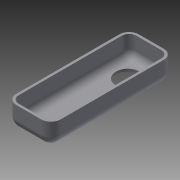
# Autodesk Inventor part: NodeMCU_MQ-4_top_shelled
Saved by Autodesk Inventor 2014 SP1 (Build 180222100, 222)
## iProperties
Created: 2016-10-27
Part Number: NodeMCU_MQ-4_top_shelled
Material: Generic
Document SubType Name: Modeling
Designer: danielsikar
Density: 1 g/cm^3
Appearance: Default
Author: danielsikar
Autodesk Inventor part; units mm, degrees
ref_plane "YZ Plane" through (0, 0, 0) normal (1, 0, 0) x (0, 1, 0)
ref_plane "XZ Plane" through (0, 0, 0) normal (0, 1, 0) x (-1, 0, 0)
ref_plane "XY Plane" through (0, 0, 0) normal (0, 0, 1) x (1, 0, 0)
sketch "Sketch1" plane through (0, 0, 0) normal (0, 0, 1) x (1, 0, 0)
  line L0 (0, 0) -> (37, 0)
  line L1 (37, 0) -> (37, 102.3)
  line L2 (37, 102.3) -> (0, 102.3)
  line L3 (0, 102.3) -> (0, 0)
  dimension "d0" = 37
  dimension "d1" = 102.3
  constraints: 8 end point, 2 parallel, 1 horizontal, 1 perpendicular
  measures "d0" distance of L2.end L1.end
  measures "d1" distance of L1.end L0.end
extrude "Extrusion1" add sketch "Sketch1" along normal blind 19
fillet "Fillet1" radius 8 4 edges at (0, 0, 9.5) (37, 0, 9.5) (37, 102.3, 9.5) (0, 102.3, 9.5)
fillet "Fillet2" radius 8 8 edges at (34.6569, 99.9569, 0) (18.5, 102.3, 0) (2.3431, 99.9569, 0) (0, 51.15, 0) (2.3431, 2.3431, 0) (18.5, 0, 0) (34.6569, 2.3431, 0) (37, 51.15, 0)
shell "Shell1" thickness 2 removed faces 1 at (12.3333, 36.7667, 19)
sketch "Sketch2" plane through (0, 0, 0) normal (0, 0, -1) x (-1, 0, 0)
  circle A0 centre (-18.5, 82.8) radius 10
  line L0 (-8, 102.3) -> (-29, 102.3) projected
  point P0 (0, 0)
  dimension "d7" = 20
  dimension "d8" = 19.5
  constraints: 1 centre point
  measures "d7" diameter of A0
  measures "d8" distance from line of A0.centre L0
extrude "Extrusion2" cut sketch "Sketch2" against normal blind 19
body "Solid1"
